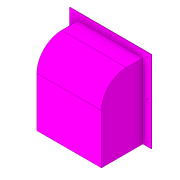
# Autodesk Inventor part: SidePanelCover-Curved
Saved by Autodesk Inventor 2017 (Build 210142000, 142)
## iProperties
Created: 2017-11-14
Part Number: SidePanelCover-Curved
Material: Generic
Document SubType Name: Modeling
Designer: Kathryn Rosie
Density: 1 g/cm^3
Appearance: Default Generic
Author: Kathryn Rosie
Autodesk Inventor part; units mm, degrees
ref_plane "YZ Plane" through (0, 0, 0) normal (1, 0, 0) x (0, 1, 0)
ref_plane "XZ Plane" through (0, 0, 0) normal (0, 1, 0) x (-1, 0, 0)
ref_plane "XY Plane" through (0, 0, 0) normal (0, 0, 1) x (1, 0, 0)
sketch "Sketch1" plane through (0, 0, 0) normal (1, 0, 0) x (0, 1, 0)
  line L0 (-225, -125) -> (225, -125)
  line L1 (225, -125) -> (225, -25)
  line L2 (75, 125) -> (-225, 125)
  line L3 (-225, 125) -> (-225, -125)
  line L4 (-225, -125) -> (225, 125) construction
  line L5 (225, -125) -> (-225, 125) construction
  arc A0 (225, -25) -> (75, 125) centre (75, -25) ccw
  point P0 (0, 0)
  dimension "d0" = 450
  dimension "d1" = 250
  dimension "d2" = 150
  constraints: 12 end point, 2 midpoint, 2 parallel, 2 point on circle, 2 point on line, 2 tangent, 1 centre point, 1 horizontal, 1 perpendicular
  measures "d0" distance of L2.end L4.end
  measures "d1" distance of L4.end L0.end
  measures "d2" radius of A0
extrude "Extrusion1" add sketch "Sketch1" along normal mid plane 390
shell "Shell1" thickness 2 removed faces 1 at (65, -75, -125)
sketch "Sketch2" plane through (195, 225, -125) normal (0, 0, -1) x (-1, 0, 0)
  line L0 (2, -448) -> (2, -2) projected
  line L1 (2, -2) -> (388, -2) projected
  line L2 (388, -2) -> (388, -448) projected
  line L3 (388, -2) -> (388, -448)
  line L4 (2, -448) -> (2, -2)
  line L5 (2, -2) -> (388, -2)
  line L6 (442, -450) -> (442, 44)
  line L7 (442, 44) -> (-52, 44)
  line L8 (-52, 44) -> (-52, -450)
  line L9 (0, -450) -> (390, -450) projected
  line L10 (2, -448) -> (2, -450)
  line L11 (388, -448) -> (388, -450)
  line L12 (-52, -450) -> (2, -450)
  line L13 (388, -450) -> (442, -450)
  point P0 (195, -225)
  point P1 (195, -450)
  dimension "d6" = 494
  dimension "d7" = 494
  constraints: 20 end point, 4 parallel, 4 perpendicular, 3 point on line, 2 horizontal, 1 midpoint
  measures "d6" distance of L6.start L6.end
  measures "d7" distance of L6.end L7.end
sketch "Sketch3" plane through (-193, -223, -125) normal (0, 1, 0) x (1, 0, 0)
  line L0 (0, 0) -> (386, 0) projected
  line L1 (0, 0) -> (0, -248) projected
  line L2 (0, -248) -> (386, -248) projected
  line L3 (386, -248) -> (386, 0) projected
  point P0 (193, -125)
extrude "Extrusion2" cut sketch "Sketch3" against normal blind 2
extrude "Extrusion3" add sketch "Sketch2" along normal blind 2 contours L10 L9 L12 L8 L7 L6 L13 L11 L2 L1 L0
hole "Hole1" at (-222, 244, -127) direction (0, 0, 1) diameter 6 end through all
pattern_linear "Rectangular Pattern1" count 3 spacing 222 along (1, 0, 0) count 3 spacing 222 along (0, -1, 0) of "Hole1"
body "Solid1"
